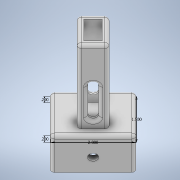
# Autodesk Inventor part: Sample Holder end for 8020-neutron-whispervalve-r2
Saved by Autodesk Inventor 2020 (Build 240168000, 168)
## iProperties
Created: 2022-02-15
Part Number: Sample Holder end for 8020-neutron-whispervalve-r2
Material: Generic
Document SubType Name: Modeling
Designer: Beaucage
Density: 1 g/cm^3
Appearance: Default
Author: Beaucage
Autodesk Inventor part; units mm, degrees
ref_plane "YZ Plane" through (0, 0, 0) normal (1, 0, 0) x (0, 1, 0)
ref_plane "XZ Plane" through (0, 0, 0) normal (0, 1, 0) x (-1, 0, 0)
ref_plane "XY Plane" through (0, 0, 0) normal (0, 0, 1) x (1, 0, 0)
sketch "Sketch1" plane through (0, 0, 0) normal (0, 1, 0) x (-1, 0, 0)
  line L0 (0, 0) -> (38.1, 0)
  line L1 (38.1, 0) -> (38.1, -50.8)
  line L2 (38.1, -50.8) -> (0, -50.8)
  line L3 (0, -50.8) -> (0, 0)
  line L4 (38.1, -50.8) -> (33.02, -50.8)
  line L5 (33.02, -50.8) -> (33.02, 0)
  line L6 (33.02, 0) -> (38.1, 0)
  line L7 (38.1, 0) -> (38.1, -50.8)
  line L8 (0, -50.8) -> (5.08, -50.8)
  line L9 (5.08, -50.8) -> (5.08, 0)
  line L10 (5.08, 0) -> (0, 0)
  line L11 (0, 0) -> (0, -50.8)
  dimension "d0" = 38.1
  dimension "d1" = 50.8
  dimension "d2" = 5.08
  dimension "d3" = 5.08
  constraints: 24 end point, 6 parallel, 3 horizontal, 3 perpendicular, 2 point on line
  measures "d0" distance of L1.end L2.end
  measures "d1" distance of L0.end L1.end
  measures "d2" distance of L5.end L6.end
  measures "d3" distance of L10.end L9.end
extrude "Extrusion1" add sketch "Sketch1" along normal blind 25.4 contours L0 L9 L2 L3 | L0 L1 L2 L5
extrude "Extrusion2" add sketch "Sketch1" against normal blind 5.08
sketch "Sketch2" plane through (0, 25.4, 0) normal (1, 0, 0) x (0, 0, -1)
  line L0 (50.8, 0) -> (0, 0) projected
  line L1 (25.4, 0) -> (25.4, -12.7)
  point P0 (0, -25.4)
  dimension "d8" = 12.7
  constraints: 2 end point, 1 midpoint, 1 vertical
  measures "d8" distance of L1.start L1.end
hole "Hole1" at (0, 12.7, -25.4) direction (-1, 0, 0) diameter 6.7564 end through all clearance for "Socket Head Cap Screw" size "1/4" standard "Ansi Unified Screw Threads"
sketch "Sketch3" plane through (0, -5.08, 0) normal (0, -1, 0) x (1, 0, 0)
  line L0 (0, 0) -> (-19.05, 0)
  line L1 (0, 0) -> (-38.1, 0) projected
  line L2 (-19.05, 0) -> (-19.05, -25.4)
  line L3 (-6, -34.85) -> (-6, -15.95)
  line L4 (-6, -15.95) -> (-32.1, -15.95)
  line L5 (-32.1, -15.95) -> (-32.1, -34.85)
  line L6 (-32.1, -34.85) -> (-6, -34.85)
  line L7 (-6, -34.85) -> (-32.1, -15.95) construction
  line L8 (-6, -15.95) -> (-32.1, -34.85) construction
  line L9 (-10, -19.95) -> (-10, -30.85)
  line L10 (-10, -30.85) -> (-28.1, -30.85)
  line L11 (-28.1, -30.85) -> (-28.1, -19.95)
  line L12 (-28.1, -19.95) -> (-10, -19.95)
  line L13 (-10, -19.95) -> (-28.1, -30.85) construction
  line L14 (-10, -30.85) -> (-28.1, -19.95) construction
  dimension "d16" = 25.4
  dimension "d17" = 18.9
  dimension "d18" = 26.1
  dimension "d19" = 10.9
  dimension "d20" = 18.1
  constraints: 28 end point, 4 parallel, 3 perpendicular, 1 midpoint
  measures "d16" distance of L0.end L2.end
  measures "d17" distance of L5.end L4.end
  measures "d18" distance of L4.end L3.end
  measures "d19" distance of L10.end L11.end
  measures "d20" distance of L9.end L10.end
extrude "Extrusion3" add sketch "Sketch3" along normal blind 69.85
sketch "Sketch4" plane through (-6, -5.08, -15.95) normal (1, 0, 0) x (0, 0, -1)
  line L0 (18.9, 0) -> (18.9, -69.85) projected
  line L1 (18.9, -34.925) -> (9.4512, -34.925)
  line L2 (9.4512, -34.925) -> (9.4512, -9.525) construction
  line L3 (12.6262, -34.925) -> (12.6262, -9.525)
  line L4 (6.2762, -9.525) -> (6.2762, -34.925)
  arc A0 (6.2762, -34.925) -> (12.6262, -34.925) centre (9.4512, -34.925) ccw
  arc A1 (12.6262, -9.525) -> (6.2762, -9.525) centre (9.4512, -9.525) ccw
  point P0 (-15.95, 5.08)
  point P1 (9.4512, -22.225)
  dimension "d23" = 9.4488
  dimension "d24" = 25.4
  dimension "d25" = 6.35
  constraints: 10 end point, 4 point on circle, 4 tangent, 2 centre point, 2 midpoint, 1 horizontal, 1 parallel, 1 vertical
  measures "d23" distance of L1.start L1.end
  measures "d24" distance of L1.end L2.end
  measures "d25" diameter of A1
extrude "Extrusion4" cut sketch "Sketch4" against normal blind 76.2
fillet "Fillet1" radius 2.54 24 edges at (-38.1, -5.08, -25.4) (0, -5.08, -25.4) (-6, -11.43, -25.4012) (-6, -27.305, -28.5762) (-6, -43.18, -25.4012) (-6, -27.305, -22.2262) (-6, -40.005, -15.95) (-6, -40.005, -34.85) (-6, -74.93, -25.4) (-19.05, -74.93, -15.95) (-19.05, -74.93, -34.85) (-32.1, -74.93, -25.4) (-32.1, -40.005, -15.95) (-32.1, -40.005, -34.85) (-32.1, -27.305, -28.5762) (-32.1, -11.43, -25.4012) (-32.1, -27.305, -22.2262) (-32.1, -43.18, -25.4012) (-19.05, -5.08, -50.8) (-38.1, 10.16, -50.8) (-38.1, 10.16, 0) (-19.05, -5.08, 0) (0, 10.16, -50.8) (0, 10.16, 0)
body "Solid1"
